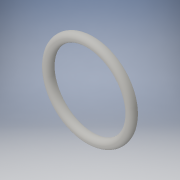
# Autodesk Inventor part: msheehan_ring_small
Saved by Autodesk Inventor 2016 (Build 200138000, 138)
## iProperties
Created: 2017-08-31
Part Number: msheehan_ring_small
Material: Generic
Document SubType Name: Modeling
Designer: Student
Density: 1 g/cm^3
Appearance: Default
Author: Student
Autodesk Inventor part; units mm, degrees
ref_plane "YZ Plane" through (0, 0, 0) normal (1, 0, 0) x (0, 1, 0)
ref_plane "XZ Plane" through (0, 0, 0) normal (0, 1, 0) x (-1, 0, 0)
ref_plane "XY Plane" through (0, 0, 0) normal (0, 0, 1) x (1, 0, 0)
sketch "Sketch1" plane through (0, 0, 0) normal (1, 0, 0) x (0, 1, 0)
  line L0 (0, 0) -> (0, -47.498)
  line L1 (0, -23.749) -> (23.749, -23.749)
  circle A0 centre (23.749, -23.749) radius 2.54
  dimension "d0" = 47.498
  dimension "d1" = 23.749
  dimension "d2" = 5.08
  constraints: 4 end point, 1 centre point, 1 coincident, 1 horizontal, 1 midpoint, 1 vertical
  measures "d0" distance of L0.start L0.end
  measures "d1" distance of L1.start L1.end
  measures "d2" diameter of A0
revolve "Revolution1" add sketch "Sketch1" angle 360 about axis through (0, 0, 0) along (0, 0, -1)
sketch "Sketch2" plane through (0, 0, 0) normal (0, 0, 1) x (1, 0, 0)
  circle A0 centre (0, 0) radius 26.289 projected
  line L0 (0, 26.289) -> (0, -26.289) construction
  circle A1 centre (0, 0) radius 26.289 projected
  dimension "d5" = 52.578
  constraints: 2 end point, 2 vertical alignment, 1 vertical, 2 other
  measures "d5" distance of L0.start L0.end
sketch "Sketch3" plane through (0, 0, 0) normal (0, 0, 1) x (1, 0, 0)
  circle A0 centre (0, 0) radius 21.209 projected
  line L0 (0, -21.209) -> (0, -26.289) construction
  circle A1 centre (0, 0) radius 26.289 projected
  dimension "d6" = 5.08
  constraints: 2 end point, 2 vertical alignment, 1 vertical, 2 other
  measures "d6" distance of L0.start L0.end
body "Solid1"
